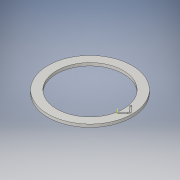
# Autodesk Inventor part: DiskCam
Saved by Autodesk Inventor 2016 (Build 200138000, 138)
## iProperties
Created: 2015-07-20
Part Number: DiskCam
Material: PC/ABS Plastic
Document SubType Name: Modeling
Designer: steele
Density: 0.357273 g/cm^3
Appearance: Smooth - White
Mass: 179.331 g
Surface Area: 1053.95 cm^2
Volume: 501.944 cm^3
Author: steele
Autodesk Inventor part; units mm, degrees
ref_plane "YZ Plane" through (0, 0, 0) normal (1, 0, 0) x (0, 1, 0)
ref_plane "XZ Plane" through (0, 0, 0) normal (0, 1, 0) x (-1, 0, 0)
ref_plane "XY Plane" through (0, 0, 0) normal (0, 0, 1) x (1, 0, 0)
sketch "Sketch1" plane through (0, 0, 0) normal (0, 1, 0) x (-1, 0, 0)
  circle A0 centre (0, 0) radius 146.05
  circle A1 centre (0, 0) radius 184.15
  dimension "camInsideDiameter" = 292.1
  dimension "d1" = 368.3
  constraints: 2 centre point, 2 coincident
  measures "camInsideDiameter" diameter of A0
  measures "d1" diameter of A1
extrude "Extrusion1" add sketch "Sketch1" along normal blind 12.7
sketch "Sketch2" plane through (0, 12.7, 0) normal (0, 1, 0) x (1, 0, 0)
  circle A0 centre (0, 0) radius 146.05 construction
  circle A1 centre (0, 0) radius 184.15 construction
  line L0 (0, 0) -> (149.4717, -29.7318) construction
  line L1 (0, 0) -> (184.15, 0) construction
  line L2 (0, 0) -> (149.4717, 29.7318) construction
  line L3 (149.4717, -29.7318) -> (171.7568, -6.3426)
  line L4 (149.4717, 29.7318) -> (171.7568, 6.3426)
  arc A2 (171.7568, -6.3426) -> (171.7568, 6.3426) centre (165.1, 0) ccw
  dimension "oneHalfPhase" = 11.25
  dimension "d5" = 11.25
  dimension "innerRadiusForCam" = 152.4
  dimension "innerRadisuForCam" = 152.4
  dimension "d12" = 165.1
  constraints: 10 end point, 2 point on circle, 2 tangent, 1 centre point, 1 horizontal, 1 horizontal alignment, 1 point on line, 1 other
  measures "oneHalfPhase" angle of L0 L1
  measures "d5" angle of L2 L1
  measures "innerRadiusForCam" distance of point (0, 0) L2.end
  measures "innerRadisuForCam" distance of L0.start L0.end
  measures "d12" distance of point (0, 0) A2.centre
ref_plane "Work Plane1" through (149.4717, 12.7, 29.7318) normal (0.6898129, 0, -0.7239876) x (0, 1, 0)
sketch "Sketch4" plane through (149.4717, 12.7, 29.7318) normal (0.6898129, 0, -0.7239876) x (0, 1, 0)
  circle A0 centre (0, 0) radius 3.175
  point P0 (-12.7, -128.725)
  dimension "d9" = 6.35
  constraints: 1 centre point
  measures "d9" diameter of A0
sweep "Sweep1" cut profiles "Sketch4" path "Sketch2" path curves L3 A2 L4
equation "\"d5\" = oneHalfPhase"
equation "\"innerRadiusForCam\" = innerRadisuForCam"
body "Solid1"
